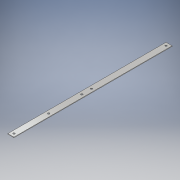
# Autodesk Inventor part: Rig
Saved by Autodesk Inventor 2019.3 (Build 233278000, 278)
## iProperties
Created: 2019-06-16
Part Number: Rig
Material: Aluminium 6061
Document SubType Name: Modeling
Designer: Jonas
Density: 2.7 g/cm^3
Appearance: Aluminium - poliert
Author: Jonas
Autodesk Inventor part; units mm, degrees
ref_plane "YZ Plane" through (0, 0, 0) normal (1, 0, 0) x (0, 1, 0)
ref_plane "XZ Plane" through (0, 0, 0) normal (0, 1, 0) x (-1, 0, 0)
ref_plane "XY Plane" through (0, 0, 0) normal (0, 0, 1) x (1, 0, 0)
sketch "Skizze1" plane through (0, 0, 0) normal (0, 1, 0) x (-1, 0, 0)
  line L0 (-7.0769, 11.8974) -> (2.9231, 11.8974)
  line L1 (2.9231, 11.8974) -> (2.9231, -250.1026)
  line L2 (2.9231, -250.1026) -> (-7.0769, -250.1026)
  line L3 (-7.0769, -250.1026) -> (-7.0769, 11.8974)
  point P0 (0, 0)
  dimension "d0" = 262
  dimension "d1" = 10
  constraints: 8 end point, 2 parallel, 1 horizontal, 1 perpendicular
  measures "d0" distance of L0.end L1.end
  measures "d1" distance of L0.start L0.end
extrude "Extrusion1" add sketch "Skizze1" along normal blind 1
sketch "Skizze2" plane through (0, 1, 0) normal (0, 1, 0) x (1, 0, 0)
  line L0 (-2.9231, -11.8974) -> (7.0769, -11.8974) projected
  line L1 (7.0769, -11.8974) -> (7.0769, 250.1026) projected
  line L2 (7.0769, 250.1026) -> (-2.9231, 250.1026) projected
  point P0 (0, 0)
  point P1 (2.0769, -6.8974)
  point P2 (2.0769, 245.1026)
  dimension "d4" = 5
  dimension "d5" = 5
  dimension "d13" = 5
  dimension "d14" = 5
  measures "d4" distance from line of point (2.077, -6.897) L0
  measures "d5" distance from line of L1 point (2.077, -6.897)
  measures "d13" distance from line of L2 point (2.077, 245.103)
  measures "d14" distance from line of L1 point (2.077, 245.103)
hole "Bohrung1" at (2.0769, 1, 6.8974) direction (0, -1, 0) diameter 3 end through all
sketch "Skizze3" plane through (0, 1, 0) normal (0, 1, 0) x (1, 0, 0)
  line L0 (7.0769, 250.1026) -> (-2.9231, 250.1026) projected
  line L1 (7.0769, -11.8974) -> (7.0769, 250.1026) projected
  point P0 (0, 0)
  point P1 (2.0769, 245.1026)
  dimension "d15" = 5
  dimension "d16" = 5
  measures "d15" distance from line of L0 point (2.077, 245.103)
  measures "d16" distance from line of L1 point (2.077, 245.103)
hole "Bohrung2" at (2.0769, 1, -245.1026) direction (0, -1, 0) diameter 3 end through all
sketch "Skizze4" plane through (0, 1, 0) normal (0, 1, 0) x (1, 0, 0)
  line L0 (-2.9231, -11.8974) -> (7.0769, -11.8974) projected
  line L1 (7.0769, -11.8974) -> (7.0769, 250.1026) projected
  line L2 (7.0769, 250.1026) -> (-2.9231, 250.1026) projected
  point P0 (0, 0)
  point P1 (2.0769, 121.6026)
  dimension "d25" = 5
  dimension "d33" = 128.5
  measures "d25" distance from line of L1 point (2.077, 121.603)
  measures "d33" distance from line of L2 point (2.077, 121.603)
hole "Bohrung3" at (2.0769, 1, -121.6026) direction (0, -1, 0) diameter 3 end through all
sketch "Skizze5" plane through (0, 1, 0) normal (0, 1, 0) x (1, 0, 0)
  line L0 (-2.9231, -11.8974) -> (7.0769, -11.8974) projected
  line L1 (7.0769, -11.8974) -> (7.0769, 250.1026) projected
  line L2 (7.0769, 250.1026) -> (-2.9231, 250.1026) projected
  point P0 (0, 0)
  point P1 (2.0769, 50.6026)
  point P2 (2.0769, 105.6026)
  dimension "d35" = 5
  dimension "d44" = 144.5
  dimension "d45" = 55
  measures "d35" distance from line of L1 point (2.077, 50.603)
  measures "d44" distance from line of L2 point (2.077, 105.603)
  measures "d45" distance of point (2.077, 50.603) point (2.077, 105.603)
hole "Bohrung4" at (2.0769, 1, -50.6026) at (2.0769, 1, -105.6026) direction (0, -1, 0) diameter 3 end through all
